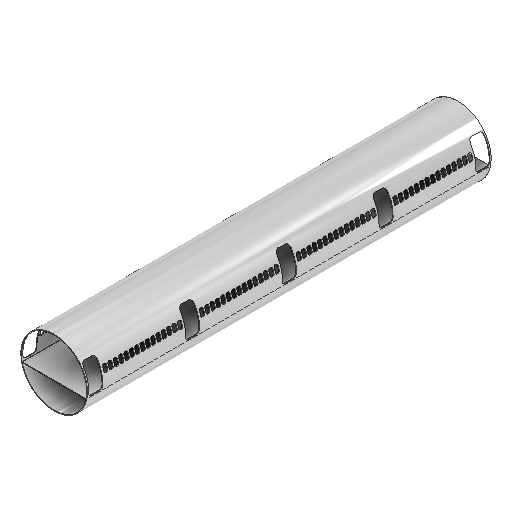
# Autodesk Inventor part: Parametric Fuselage
Saved by Autodesk Inventor 2026.2 (Build 302298000, 298)
## iProperties
Created: 2026-01-29
Part Number: Parametric Fuselage
Material: Generic
Document SubType Name: Modeling
Designer: andyeske
Density: 1 g/cm^3
Appearance: Default
Author: andyeske
Autodesk Inventor part; units mm, degrees
ref_plane "XZ Plane" through (0, 0, 0) normal (0, 1, 0) x (-1, 0, 0)
sketch "Sketch1" plane through (0, 0, 0) normal (0, 0, 1) x (1, 0, 0)
  circle A0 centre (0, 0) radius 12.7
  circle A1 centre (0, 0) radius 12.446
  line L0 (-12.1841, -2.54) -> (12.1841, -2.54)
  line L1 (-12.1283, -2.794) -> (12.1283, -2.794)
  dimension "d0" = 25.4
  dimension "d1" = 0.254
  dimension "d2" = 2.54
  dimension "d3" = 0.254
  constraints: 4 end point, 4 point on circle, 2 centre point, 2 horizontal, 1 coincident
  measures "d0" diameter of A0
  measures "d1" radial gap between concentric circles of A0 A1
  measures "d2" distance from line of L0 point (0, 0)
  measures "d3" distance between parallel lines of L0 L1
extrude "Extrusion1" add sketch "Sketch1" along normal blind 43.18 contours A0 | L0 A1 L1
ref_plane "Work Plane1" through (50.8, 0, 0) normal (1, 0, 0) x (0, 1, 0)
sketch "Sketch2" plane through (50.8, 0, 0) normal (1, 0, 0) x (0, 1, 0)
  line L0 (12.7, 43.18) -> (-12.7, 43.18) construction
  line L1 (12.7, 0) -> (-12.7, 0) construction
  line L2 (-2.54, 43.18) -> (-2.54, 0) construction
  line L3 (12.7, 43.18) -> (12.7, 36.83) construction
  line L4 (12.7, 36.83) -> (-2.54, 36.83) construction
  line L5 (12.7, 36.83) -> (12.7, 34.798) construction
  line L6 (12.7, 34.798) -> (-2.54, 34.798) construction
  line L7 (8.128, 42.672) -> (-2.032, 42.672)
  line L8 (-2.032, 42.672) -> (-2.032, 37.338)
  line L9 (-2.032, 37.338) -> (8.128, 37.338)
  line L10 (8.128, 37.338) -> (8.128, 42.672)
  line L11 (5.08, 36.576) -> (2.54, 36.576)
  line L12 (2.54, 36.576) -> (2.54, 35.052)
  line L13 (2.54, 35.052) -> (5.08, 35.052)
  line L14 (5.08, 35.052) -> (5.08, 36.576)
  point P0 (0, 0)
  point P1 (3.81, 35.052)
  dimension "d7" = 6.35
  dimension "d8" = 2.032
  dimension "d9" = 0.508
  dimension "d10" = 0.508
  dimension "d11" = 0.508
  dimension "d12" = 5.08
  dimension "d13" = 0.254
  dimension "d14" = 0.254
  dimension "d15" = 2.54
  dimension "d16" = 10.16
  constraints: 26 end point, 5 perpendicular, 4 parallel, 3 point on line, 2 horizontal, 2 vertical, 1 midpoint
  measures "d7" distance between parallel lines of L0 L4
  measures "d8" distance of L3.end L5.end
  measures "d9" distance between parallel lines of L0 L7
  measures "d10" distance between parallel lines of L4 L9
  measures "d11" distance between parallel lines of L2 L8
  measures "d12" distance between parallel lines of L2 L12
  measures "d13" distance between parallel lines of L4 L11
  measures "d14" distance from line of L6 point (3.81, 35.052)
  measures "d15" distance of L12.end L13.end
  measures "d16" distance of L7.start L7.end
emboss "Emboss1" sketch "Sketch2" operation cut depth 0.254 direction (-1, 0, 0) contours L10 L9 L8 L7
fillet "Fillet1" radius 1.27 4 edges at (12.4077, -2.032, 37.338) (12.4077, -2.032, 42.672) (9.5919, 8.128, 42.672) (9.5919, 8.128, 37.338)
emboss "Emboss2" sketch "Sketch2" operation cut depth 2.54 direction (-1, 0, 0) contours L14 L13 L12 L11
fillet "Fillet2" radius 0.508 4 edges at (11.5009, 5.08, 36.576) (11.5009, 5.08, 35.052) (12.3137, 2.54, 35.052) (12.3137, 2.54, 36.576)
pattern_linear "Rectangular Pattern1" count 15 spacing 2.032 along (0, 0, -1) of "Emboss2", "Fillet2"
ref_plane "Work Plane2" through (0, 0, 21.59) normal (0, 0, 1) x (1, 0, 0)
mirror "Mirror1" about plane through (0, 0, 21.59) normal (0, 0, 1) of "Emboss1", "Fillet1"
sketch "Sketch4" plane through (0, 0, 0) normal (1, 0, 0) x (0, 1, 0)
  line L0 (29.9989, 66.0716) -> (-27.1376, 66.0716)
  line L1 (-27.1376, 66.0716) -> (-27.1376, -50.701)
  line L2 (-27.1376, -50.701) -> (29.9989, -50.701)
  line L3 (29.9989, -50.701) -> (29.9989, 66.0716)
  point P0 (0, 0)
  constraints: 8 end point, 2 parallel, 1 horizontal, 1 perpendicular
extrude "Extrusion2" cut sketch "Sketch4" against normal blind 55.88
pattern_linear "Rectangular Pattern2" count 4 spacing 36.83 along (0, 0, 1)
mirror "Mirror2" about plane through (0, 1.4306, 7.6853) normal (-1, 0, 0)
equation "\"d0\" = Diameter"
equation "\"d1\" = 0.01 * Diameter"
equation "\"d3\" = 0.01 * Diameter"
equation "\"d12\" = 0.2 * Diameter"
equation "\"d15\" = 0.1 * Diameter"
equation "\"d16\" = 0.4 * Diameter"
equation "\"d2\" = 0.1 * Diameter"
equation "\"d26\" = 2.032 * N_Windows + 6.35 * N_Exits"
equation "\"Diameter\" = 25.4"
equation "\"N_Windows\" = 15"
equation "\"N_Exits\" = 4"
body "Solid1"
